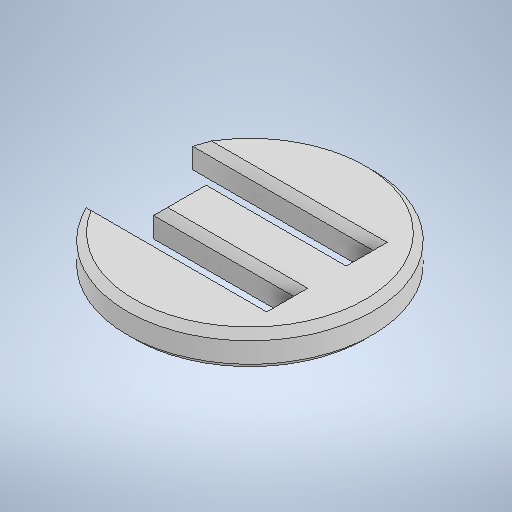
# Autodesk Inventor part: Clips
Saved by Autodesk Inventor 2026.2 (Build 302298010, 298A)
## iProperties
Created: 2026-05-07
Part Number: Clips
Material: Generic
Document SubType Name: Modeling
Designer: piete
Density: 1 g/cm^3
Appearance: Default
Author: piete
Autodesk Inventor part; units mm, degrees
ref_plane "YZ Plane" through (0, 0, 0) normal (1, 0, 0) x (0, 1, 0)
ref_plane "XZ Plane" through (0, 0, 0) normal (0, 1, 0) x (-1, 0, 0)
ref_plane "XY Plane" through (0, 0, 0) normal (0, 0, 1) x (1, 0, 0)
sketch "Sketch1" plane through (0, 0, 0) normal (0, 1, 0) x (-1, 0, 0)
  line L0 (10, 3.75) -> (-10, 3.75)
  line L1 (-10, 3.75) -> (-10, -3.75)
  line L2 (-10, -3.75) -> (10, -3.75)
  line L3 (10, -3.75) -> (10, 3.75)
  line L4 (10, 7.6) -> (-10, 7.6)
  line L5 (-10, 7.6) -> (-10, -7.6)
  line L6 (-10, -7.6) -> (10, -7.6)
  line L7 (10, -7.6) -> (10, 7.6)
  circle A0 centre (0, 0) radius 17.5
  line L8 (10, -7.6) -> (15.7636, -7.6)
  line L9 (10, 7.6) -> (15.7636, 7.6)
  dimension "d1" = 20
  dimension "d2" = 7.5
  dimension "d3" = 20
  dimension "d4" = 15.2
  dimension "d5" = 7.6
  dimension "d6" = 3.75
  dimension "d7" = 10
  dimension "d8" = 10
  dimension "d9" = 35
  constraints: 20 end point, 5 parallel, 3 horizontal, 2 perpendicular, 2 point on circle, 1 centre point, 1 coincident
  measures "d1" distance of L2.end L1.end
  measures "d2" distance of L1.end L0.end
  measures "d3" distance of L6.end L5.end
  measures "d4" distance of L5.end L4.end
  measures "d5" distance from line of point (0, 0) L6
  measures "d6" distance from line of point (0, 0) L2
  measures "d7" distance from line of point (0, 0) L5
  measures "d8" distance from line of point (0, 0) L1
  measures "d9" diameter of A0
extrude "Extrusion1" add sketch "Sketch1" along normal blind 4.9 contours L3 L2 L1 L0 | L1 L5 L6 L8 A0 L9 L4
chamfer "Chamfer1" distance 1 angle 45 16 edges at (-10, 4.9, 0) (0, 4.9, 3.75) (0, 4.9, -3.75) (10, 4.9, -5.675) (0, 4.9, -7.6) (17.5, 4.9, 0) (0, 4.9, 7.6) (10, 4.9, 5.675) (17.5, 0, 0) (0, 0, -7.6) (0, 0, -3.75) (0, 0, 3.75) (0, 0, 7.6) (10, 0, 5.675) (10, 0, -5.675) (-10, 0, 0)
equation "\"d5\" = 0.5 * d4"
equation "\"d6\" = 0.5 * d2"
equation "\"d7\" = 0.5 * d3"
equation "\"d8\" = 0.5 * d1"
body "Solid1"
